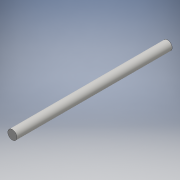
# Autodesk Inventor part: Lifting Shaft
Saved by Autodesk Inventor 2016 (Build 200138000, 138)
## iProperties
Created: 2016-04-14
Part Number: Lifting Shaft
Material: Generic
Document SubType Name: Modeling
Designer: Spencer
Density: 1 g/cm^3
Appearance: Default
Author: Spencer
Autodesk Inventor part; units mm, degrees
ref_plane "YZ Plane" through (0, 0, 0) normal (1, 0, 0) x (0, 1, 0)
ref_plane "XZ Plane" through (0, 0, 0) normal (0, 1, 0) x (-1, 0, 0)
ref_plane "XY Plane" through (0, 0, 0) normal (0, 0, 1) x (1, 0, 0)
sketch "Sketch1" plane through (0, 0, 0) normal (0, 1, 0) x (-1, 0, 0)
  circle A0 centre (0, 0) radius 4.8
  dimension "d0" = 9.6
  constraints: 1 centre point, 1 coincident
  measures "d0" diameter of A0
extrude "Extrusion1" add sketch "Sketch1" along normal blind 162
sketch "Sketch2" plane through (0, 162, 0) normal (0, 1, 0) x (1, 0, 0)
  line L0 (-3.8312, -2.1) -> (3.8312, -2.1)
  line L1 (3.8312, -2.1) -> (3.8312, 2.1)
  line L2 (3.8312, 2.1) -> (-3.8312, 2.1)
  line L3 (-3.8312, 2.1) -> (-3.8312, -2.1)
  line L4 (-3.8312, -2.1) -> (3.8312, 2.1) construction
  line L5 (3.8312, -2.1) -> (-3.8312, 2.1) construction
  arc A0 (-3.8312, 2.1) -> (-3.8312, -2.1) centre (-0.4025, 0) ccw
  line L6 (-4.4232, 0) -> (-3.8312, 0)
  line L7 (3.8312, 0) -> (4.4232, 0)
  arc A1 (3.8312, -2.1) -> (3.8312, 2.1) centre (0.4025, 0) ccw
  circle A2 centre (0, 0) radius 4.8 projected
  line L8 (-4.8, 0) -> (-4.4232, 0)
  line L9 (4.4232, 0) -> (4.8, 0)
  dimension "d3" = 0.592
  dimension "d6" = 4.2
  constraints: 20 end point, 8 point on circle, 4 midpoint, 2 centre point, 2 horizontal, 2 parallel, 2 point on line, 1 collinear, 1 perpendicular
  measures "d3" distance of L7.start L7.end
  measures "d6" distance of L2.end L0.start
extrude "Extrusion2" cut sketch "Sketch2" against normal blind 7 contours L3 L2 L1 L0 | A0 L6 L3 | L1 L7 A1 | L6 A0 L3 | L1 A1 L7
body "Solid1"
